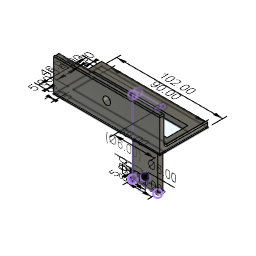
camera_holder (Autodesk Fusion 360 design; units mm, degrees)
Autodesk Fusion 360 part; units mm, degrees
sketch "Sketch1" plane through (0, 0, 0) normal (0, 0, 1) x (1, 0, 0)
sketch "Sketch2" plane through (0, 0, 0) normal (0, 0, 1) x (1, 0, 0)
  line L0 (0, 0) -> (24, 0)
  line L1 (24, 0) -> (24, 5)
  line L2 (24, 5) -> (0, 5)
  line L3 (0, 5) -> (0, 0)
  dimension "d157" = 24
  dimension "d158" = 5
  constraint horizontal L0
  constraint vertical L1
  constraint horizontal L2
  constraint vertical L3
  constraint coincident L0.start L3.end
  measures "d157" distance of L0.start L0.end
  measures "d158" distance of L0.start L2.end
extrude "Extrude1" add sketch "Sketch2" along normal blind 70
sketch "Sketch3" plane through (0, 0, 0) normal (0, -1, 0) x (1, 0, 0)
  circle A0 centre (12, 8) radius 3
  line L0 (0, 0) -> (24, 0)
  line L1 (0, 0) -> (0, 70)
  dimension "d161" = 6
  dimension "d162" = 8
  dimension "d163" = 12
  measures "d161" diameter of A0
  measures "d162" distance of A0.centre L0
  measures "d163" distance of A0.centre L1
extrude "Extrude2" cut sketch "Sketch3" against normal blind 5
sketch "Sketch4" plane through (0, 0, 0) normal (0, -1, 0) x (1, 0, 0)
sketch "Sketch5" plane through (0, 0, 0) normal (0, -1, 0) x (1, 0, 0)
  circle A0 centre (12, 8) radius 3
  dimension "d166" = 6
  measures "d166" diameter of A0
sketch "Sketch6" plane through (0, 0, 70) normal (0, 0, 1) x (-1, 0, 0)
  line L0 (39, -9) -> (-63, -9)
  line L1 (-63, -9) -> (-63, 37)
  line L2 (-63, 37) -> (39, 37)
  line L3 (39, 37) -> (39, -9)
  line L4 (-24, 0) -> (-24, -5)
  line L5 (-24, -5) -> (0, -5)
  line L6 (33, 4) -> (-57, 4)
  line L7 (-57, 4) -> (-57, 24)
  line L8 (-57, 24) -> (33, 24)
  line L9 (33, 24) -> (33, 4)
  line L10 (0, 0) -> (-24, 0)
  line L11 (39, 32) -> (-63, 32)
  dimension "d167" = 102
  dimension "d168" = 46
  dimension "d169" = 39
  dimension "d170" = 4
  dimension "d171" = 90
  dimension "d172" = 20
  dimension "d173" = 4
  dimension "d174" = 6
  dimension "d175" = 5
  constraint horizontal L0
  constraint vertical L1
  constraint horizontal L2
  constraint vertical L3
  constraint horizontal L6
  constraint vertical L7
  constraint horizontal L8
  constraint vertical L9
  constraint coincident L3 L11.start
  constraint coincident L1 L11.end
  constraint perpendicular L1 L11
  measures "d167" distance of L0.start L0.end
  measures "d168" distance of L0.start L2.end
  measures "d169" distance of L1 L4
  measures "d170" distance of L0 L5
  measures "d171" distance of L6.start L6.end
  measures "d172" distance of L6.start L8.end
  measures "d173" distance of L6 L10
  measures "d174" distance of L3 L9
  measures "d175" distance of L2 L11
extrude "Extrude3" add sketch "Sketch6" along normal blind 5 contours L0 L1 L3 L11
extrude "Extrude4" add sketch "Sketch6" along normal blind 32 contours L1 L2 L3 L11
fillet "Fillet1" radius 2 1 edges at (12, -32, 75)
fillet "Fillet2" radius 1 14 edges at (12, -37, 102) (12, -32, 102) (63, -34.5, 102) (-39, -34.5, 102) (-39, -10.5, 75) (-39, -31.4142, 75.5858) (-39, -32, 89.5) (12, -37, 70) (63, -14, 70) (12, 9, 70) (12, 9, 75) (63, -32, 89.5) (63, -31.4142, 75.5858) (63, -10.5, 75)
sketch "Sketch7" plane through (0, -32, 0) normal (0, 1, 0) x (-1, 0, 0)
  circle A0 centre (-12, 89.7801) radius 3.675
  line L0 (39, 77) -> (39, 101)
  dimension "d184" = 7.35
  dimension "d185" = 51
  measures "d184" diameter of A0
  measures "d185" distance of A0.centre L0
extrude "Extrude5" cut sketch "Sketch7" against normal blind 5
equation "d163 = d157 / 2"
